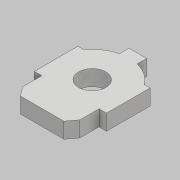
# Autodesk Inventor part: encoder_coarse
Saved by Autodesk Inventor 2017 (Build 210142000, 142)
## iProperties
Created: 2018-06-07
Part Number: encoder_coarse
Material: Generic
Document SubType Name: Modeling
Designer: Nic
Density: 1 g/cm^3
Appearance: Default
Author: Nic
Autodesk Inventor part; units mm, degrees
ref_plane "YZ Plane" through (0, 0, 0) normal (1, 0, 0) x (0, 1, 0)
ref_plane "XZ Plane" through (0, 0, 0) normal (0, 1, 0) x (-1, 0, 0)
ref_plane "XY Plane" through (0, 0, 0) normal (0, 0, 1) x (1, 0, 0)
sketch "Sketch1" plane through (0, 0, 0) normal (0, 0, 1) x (1, 0, 0)
  circle A0 centre (0, 0) radius 2
  line L0 (-5.3, 3.2) -> (-5.3, -3.2)
  line L1 (-5.3, -3.2) -> (-4.2, -3.2)
  line L2 (-4.2, -3.2) -> (-4.2, -6)
  line L3 (-4.2, -6) -> (-3.2, -7.35)
  line L4 (-3.2, -7.35) -> (0, -7.35)
  line L5 (-1.3, 6.7) -> (-1.3, 5.3)
  line L6 (-1.3, 6.7) -> (0, 6.7)
  line L7 (0, 5.3) -> (0, -7.35) construction
  arc A1 (-1.3, 5.3) -> (-4.4204, 3.2) centre (0, 0) ccw
  line L8 (-5.3, 3.2) -> (-4.4204, 3.2)
  line L9 (0, 0) -> (-5.3, 0) construction
  line L10 (5.3, 3.2) -> (5.3, -3.2)
  line L11 (5.3, -3.2) -> (4.2, -3.2)
  line L12 (4.2, -3.2) -> (4.2, -6)
  line L13 (4.2, -6) -> (3.2, -7.35)
  line L14 (3.2, -7.35) -> (0, -7.35)
  line L15 (1.3, 6.7) -> (1.3, 5.3)
  line L16 (1.3, 6.7) -> (0, 6.7)
  arc A2 (4.4204, 3.2) -> (1.3, 5.3) centre (0, 0) ccw
  line L17 (5.3, 3.2) -> (4.4204, 3.2)
  line L18 (0, 0) -> (5.3, 0) construction
  dimension "d0" = 4
  dimension "d1" = 1.3
  dimension "d2" = 5.3
  dimension "d3" = 6.7
  dimension "d4" = 4.2
  dimension "d5" = 5.3
  dimension "d7" = 3.2
  dimension "d9" = 7.35
  dimension "d10" = 3.2
  dimension "d11" = 2.8
  constraints: 38 end point, 9 symmetric about line, 4 coincident, 4 point on circle, 3 centre point, 3 horizontal, 2 midpoint, 2 perpendicular, 1 horizontal alignment, 1 parallel, 1 point on line, 1 vertical, 1 vertical alignment, 2 other
  measures "d0" diameter of A0
  measures "d1" distance of L5.start L6.end
  measures "d2" distance of point (0, 0) L7.start
  measures "d3" distance from line of point (0, 0) L6
  measures "d4" distance between parallel lines of L7 L2
  measures "d5" distance between parallel lines of L7 L0
  measures "d7" distance from line of point (0, 0) L8
  measures "d9" distance from line of L4 point (0, 0)
  measures "d10" distance of L3.end L4.end
  measures "d11" distance of L1.end L2.end
extrude "Extrusion1" add sketch "Sketch1" along normal blind 2.3
body "Solid1"
